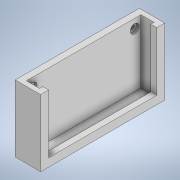
# Autodesk Inventor part: License Plate Holder
Saved by Autodesk Inventor 2022.2 (Build 262287010, 287A)
## iProperties
Created: 2022-06-18
Part Number: License Plate Holder
Material: Generic
Document SubType Name: Modeling
Designer: Main Account
Density: 1 g/cm^3
Appearance: Default
Author: Main Account
Autodesk Inventor part; units mm, degrees
ref_plane "YZ Plane" through (0, 0, 0) normal (1, 0, 0) x (0, 1, 0)
ref_plane "XZ Plane" through (0, 0, 0) normal (0, 1, 0) x (-1, 0, 0)
ref_plane "XY Plane" through (0, 0, 0) normal (0, 0, 1) x (1, 0, 0)
sketch "Sketch1" plane through (0, 0, 0) normal (1, 0, 0) x (0, 1, 0)
  circle A0 centre (0, 0) radius 3.9624 construction
  line L0 (3.9624, 0) -> (8.9624, 0) construction
  line L1 (0, 3.9624) -> (0, 10.9624) construction
  circle A1 centre (0, -101.9002) radius 3.9624 construction
  line L2 (3.9624, -101.9002) -> (8.9624, -101.9002) construction
  line L3 (0, -105.8626) -> (0, -112.8626) construction
  line L4 (8.9624, -112.8626) -> (-57.7126, -112.8626)
  line L5 (-57.7126, -112.8626) -> (-57.7126, 10.9624)
  line L6 (-57.7126, 10.9624) -> (8.9624, 10.9624)
  line L7 (8.9624, 10.9624) -> (8.9624, -112.8626)
  dimension "d0" = 7.9248
  dimension "d1" = 5
  dimension "d13" = 7
  dimension "d15" = 7.9248
  dimension "d16" = 5
  dimension "d17" = 7
  constraints: 16 end point, 4 point on circle, 3 coincident, 3 horizontal, 2 centre point, 2 parallel, 2 vertical, 1 perpendicular
  measures "d0" diameter of A0
  measures "d1" distance of L0.start L0.end
  measures "d13" distance of L1.start L1.end
  measures "d15" diameter of A1
  measures "d16" distance of L2.start L2.end
  measures "d17" distance of L3.start L3.end
extrude "Back plate" add sketch "Sketch1" along normal blind 6.35
sketch "Sketch5" plane through (6.35, 0, 0) normal (1, 0, 0) x (0, 0, -1)
  circle A0 centre (101.9002, 0) radius 3.9624 projected
  circle A1 centre (0, 0) radius 3.9624 projected
hole "Screw holes" at (6.35, 0, 0) at (6.35, 0, -101.9002) direction (-1, 0, 0) diameter 4.318 end through all counterbore diameter 8.89 counterbore depth 2.54
sketch "Sketch3" plane through (6.35, 0, 0) normal (1, 0, 0) x (0, 0, -1)
  line L0 (-10.9624, 8.9624) -> (-6.1999, 8.9624) construction
  line L1 (-10.9624, 8.9624) -> (-10.9624, -57.7126) projected
  line L2 (-6.1999, 8.9624) -> (-10.9624, 8.9624)
  line L3 (-10.9624, 8.9624) -> (-10.9624, -57.7126)
  line L4 (-10.9624, -57.7126) -> (-6.1999, -57.7126)
  line L5 (-6.1999, -57.7126) -> (-6.1999, 8.9624)
  line L6 (112.8626, -57.7126) -> (112.8626, 8.9624) projected
  line L7 (112.8626, 8.9624) -> (108.1001, 8.9624) construction
  line L8 (108.1001, 8.9624) -> (112.8626, 8.9624)
  line L9 (112.8626, 8.9624) -> (112.8626, -57.7126)
  line L10 (112.8626, -57.7126) -> (108.1001, -57.7126)
  line L11 (108.1001, -57.7126) -> (108.1001, 8.9624)
  line L12 (-6.1999, -54.5376) -> (108.1001, -54.5376)
  line L13 (108.1001, -54.5376) -> (108.1001, -57.7126)
  line L14 (108.1001, -57.7126) -> (-6.1999, -57.7126)
  point P0 (0, 0)
  point P1 (112.8626, 8.9624)
  dimension "d21" = 4.7625
  dimension "d22" = 4.7625
  dimension "d23" = 3.175
  constraints: 26 end point, 5 parallel, 3 horizontal, 3 perpendicular, 1 point on line
  measures "d21" distance of L0.start L0.end
  measures "d22" distance of L6.end L7.end
  measures "d23" distance of L4.end L12.start
extrude "Sides and bottom" add sketch "Sketch3" along normal blind 19.05
sketch "Sketch4" plane through (6.35, -54.5376, 6.1999) normal (0, 0, -1) x (-1, 0, 0)
  line L0 (0, 63.5) -> (-19.05, 63.5) construction
  line L1 (0, 0) -> (-19.05, 0) projected
  line L2 (-19.05, 0) -> (-13.208, 0)
  line L3 (-13.208, 0) -> (-13.208, 63.5)
  line L4 (-13.208, 63.5) -> (-19.05, 63.5)
  line L5 (-19.05, 63.5) -> (-19.05, 0)
  point P0 (6.35, 54.5376)
  dimension "d28" = 5.842
  constraints: 8 end point, 2 parallel, 1 horizontal, 1 perpendicular, 1 point on line
  measures "d28" distance of L0.end L3.end
extrude "Left lip" add sketch "Sketch4" along normal blind 3.175
sketch "Sketch6" plane through (6.35, -54.5376, -108.1001) normal (0, 0, 1) x (1, 0, 0)
  line L0 (19.05, 63.5) -> (19.05, 0) construction
  line L1 (19.05, 63.5) -> (13.208, 63.5) construction
  line L2 (0, 63.5) -> (19.05, 63.5) construction
  line L3 (19.05, 0) -> (13.208, 0)
  line L4 (13.208, 0) -> (13.208, 63.5)
  line L5 (13.208, 63.5) -> (19.05, 63.5)
  line L6 (19.05, 63.5) -> (19.05, 0)
  point P0 (-6.35, 54.5376)
  dimension "d38" = 5.842
  constraints: 10 end point, 2 parallel, 1 horizontal, 1 perpendicular, 1 point on line
  measures "d38" distance of L0.start L1.end
extrude "Right lip" add sketch "Sketch6" along normal blind 3.175
sketch "Sketch7" plane through (6.35, -54.5376, 6.1999) normal (0, 1, 0) x (1, 0, 0)
  line L0 (13.208, 0) -> (13.208, 3.175) projected
  line L1 (13.208, 3.175) -> (19.05, 3.175)
  line L2 (19.05, 3.175) -> (19.05, 111.125)
  line L3 (19.05, 111.125) -> (13.208, 111.125)
  line L4 (13.208, 111.125) -> (13.208, 3.175)
  point P0 (-6.35, 6.1999)
  constraints: 8 end point, 2 parallel, 1 horizontal, 1 perpendicular
extrude "Bottom lip" add sketch "Sketch7" along normal blind 5
body "Solid1"
